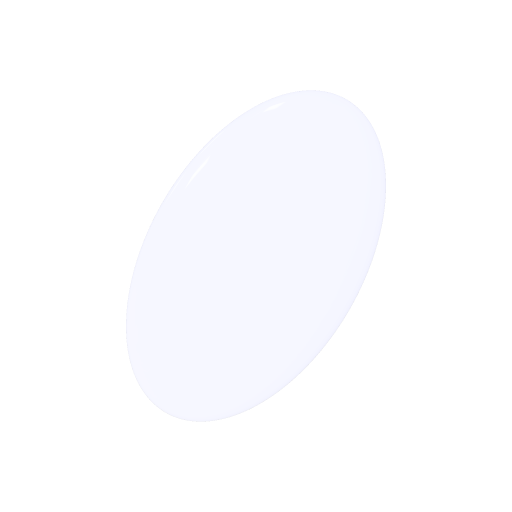
# Autodesk Inventor part: ellipse5
Saved by Autodesk Inventor 2023 (Build 270158000, 158)
## iProperties
Created: 2022-08-08
Part Number: ellipse5
Material: Generic
Document SubType Name: Modeling
Designer: Derm
Density: 1 g/cm^3
Appearance: Clear - Blue
Author: Derm
Autodesk Inventor part; units mm, degrees
ref_plane "YZ Plane" through (0, 0, 0) normal (1, 0, 0) x (0, 1, 0)
ref_plane "XZ Plane" through (0, 0, 0) normal (0, 1, 0) x (-1, 0, 0)
ref_plane "XY Plane" through (0, 0, 0) normal (0, 0, 1) x (1, 0, 0)
sketch "Sketch1" plane through (0, 0, 0) normal (0, 0, 1) x (1, 0, 0)
  ellipse E0 centre (0, 0) end of major axis (0, 1100) minor radius 200
  line L0 (-200, 0) -> (200, 0)
  dimension "d0" = 200
  dimension "d1" = 1100
  constraints: 2 end point, 1 coincident, 1 horizontal, 4 other
revolve "Revolution1" add sketch "Sketch1" angle 360 about axis through (-200, 0, 0) along (1, 0, 0) picked at (-64.5825, 220.2393) contours E0 L0
body "Solid1"
